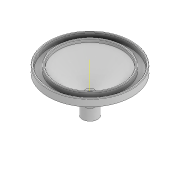
# Autodesk Inventor part: Drain Funnel v0.6.2
Saved by Autodesk Inventor 2022 (Build 260153000, 153)
## iProperties
Created: 2023-06-05
Part Number: Drain Funnel v0.6.2
Material: Generic
Document SubType Name: Modeling
Designer: cheap
Density: 1 g/cm^3
Appearance: Default
Author: cheap
Autodesk Inventor part; units mm, degrees
ref_plane "YZ Plane" through (0, 0, 0) normal (1, 0, 0) x (0, 1, 0)
ref_plane "XZ Plane" through (0, 0, 0) normal (0, 1, 0) x (-1, 0, 0)
ref_plane "XY Plane" through (0, 0, 0) normal (0, 0, 1) x (1, 0, 0)
sketch "Sketch1" plane through (0, 0, 0) normal (0, 0, 1) x (1, 0, 0)
  line L0 (0, -91.8925) -> (0, 152.1979) construction
  line L1 (3.18, 0) -> (7.58, 0)
  line L2 (7.58, 0) -> (7.58, 20)
  line L3 (7.58, 20) -> (3.18, 20)
  line L4 (3.18, 0) -> (3.18, 20)
  point P0 (0, 0)
  dimension "d1" = 3.18
  dimension "d2" = 20
  dimension "d17" = 4.4
  dimension "d18" = 7.58
  constraints: 10 end point, 3 vertical, 1 horizontal, 1 perpendicular
  measures "d1" distance of L1.start point (0, 0)
  measures "d2" distance of L1.end L2.end
  measures "d17" distance between parallel lines of L2 L4
  measures "d18" distance from line of point (0, 0) L2
revolve "Revolution1" add sketch "Sketch1" angle 360 about axis through (0, -91.8925, 0) along (0, 1, 0)
sketch "Sketch2" plane through (0, 0, 0) normal (0, 0, 1) x (1, 0, 0)
  line L0 (3.18, 0) -> (3.18, 20) projected
  line L1 (-7.58, 20) -> (7.58, 20) construction
  line L2 (7.58, 20) -> (42.58, 20) construction
  line L3 (7.58, 20) -> (7.58, 0) projected
  line L4 (38.7358, 38.6122) -> (39.7358, 38.6122)
  line L5 (38.7358, 38.6122) -> (33.7358, 38.6122)
  line L6 (39.7358, 38.6122) -> (39.7358, 43.6122)
  line L7 (33.7358, 38.6122) -> (33.7358, 43.6122)
  line L8 (39.7358, 43.6122) -> (41.7358, 43.6122)
  line L9 (41.7358, 43.6122) -> (41.7358, 36.6122)
  line L10 (41.7358, 36.6122) -> (7.58, 11.215)
  line L11 (33.7358, 43.6122) -> (31.7358, 43.6122)
  line L12 (3.18, 20) -> (7.58, 20)
  line L13 (7.58, 11.215) -> (7.58, 20)
  line L14 (0, 30.8602) -> (0, -63.1044)
  line L15 (31.7358, 43.6122) -> (31.7358, 40.4576)
  line L16 (31.7358, 40.4576) -> (3.18, 20)
  point P0 (0, 0)
  dimension "d6" = 35
  dimension "d7" = 1
  dimension "d8" = 5
  dimension "d9" = 5
  dimension "d10" = 5
  dimension "d11" = 2
  dimension "d12" = 7
  dimension "d13" = 2
  constraints: 28 end point, 5 horizontal, 3 vertical, 2 collinear, 1 parallel, 1 perpendicular, 1 point on line
  measures "d6" distance of L1.end L2.end
  measures "d7" distance of L4.start L4.end
  measures "d8" distance of L4.start L5.end
  measures "d9" distance of L4.end L6.end
  measures "d10" distance of L5.end L7.end
  measures "d11" distance of L6.end L8.end
  measures "d12" distance of L8.end L9.end
  measures "d13" distance of L7.end L11.end
revolve "Revolution2" add sketch "Sketch2" angle 360 about axis through (0, 30.8602, 0) along (0, -1, 0)
fillet "Fillet1" radius 2 1 edges at (-3.18, 20, 0)
fillet "Fillet2" radius 0.5 4 edges at (-31.7358, 43.6122, 0) (-33.7358, 43.6122, 0) (-39.7358, 43.6122, 0) (-41.7358, 43.6122, 0)
body "Solid1"
